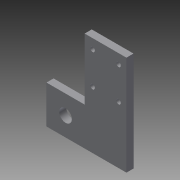
# Autodesk Inventor part: el torro bracket
Saved by Autodesk Inventor 2014 SP1 (Build 180222100, 222)
## iProperties
Created: 2014-02-18
Part Number: el torro bracket
Material: Generic
Document SubType Name: Modeling
Designer: rennoldson eimile
Density: 1 g/cm^3
Appearance: Default
Author: rennoldson eimile
Autodesk Inventor part; units mm, degrees
ref_plane "YZ Plane" through (0, 0, 0) normal (1, 0, 0) x (0, 1, 0)
ref_plane "XZ Plane" through (0, 0, 0) normal (0, 1, 0) x (-1, 0, 0)
ref_plane "XY Plane" through (0, 0, 0) normal (0, 0, 1) x (1, 0, 0)
sketch "Sketch1" plane through (0, 0, 0) normal (0, 0, 1) x (1, 0, 0)
  line L0 (-103.3855, 35.2163) -> (-23.0707, 35.2163)
  line L1 (-23.0707, 35.2163) -> (-23.0707, -64.7835)
  line L2 (-23.0707, -64.7835) -> (-103.3855, -64.7835)
  line L3 (-103.3855, -64.7835) -> (-103.3855, 35.2163)
  dimension "d0" = 80.3148
  dimension "d1" = 99.9998
  constraints: 8 end point, 2 parallel, 1 horizontal, 1 perpendicular
  measures "d0" distance of L1.end L2.end
  measures "d1" distance of L0.end L1.end
extrude "Extrusion1" add sketch "Sketch1" along normal blind 7.1628
sketch "Sketch2" plane through (0, 0, 7.1628) normal (0, 0, 1) x (1, 0, 0)
  line L0 (-23.0707, 35.2163) -> (-103.3855, 35.2163) projected
  line L1 (-103.3855, 35.2163) -> (-103.3855, -64.7835) projected
  line L2 (-103.3855, -64.7835) -> (-23.0707, -64.7835) projected
  line L3 (-23.0707, -64.7835) -> (-23.0707, 35.2163) projected
  line L4 (-65.0315, 35.2163) -> (-65.0315, -26.5819)
  line L5 (-103.3855, -26.5819) -> (-65.0315, -26.5819)
  dimension "d4" = 41.9608
  dimension "d5" = 38.2016
  constraints: 4 end point, 2 point on line, 1 parallel, 1 perpendicular
  measures "d4" distance between parallel lines of L4 L3
  measures "d5" distance between parallel lines of L5 L2
extrude "Extrusion2" cut sketch "Sketch2" against normal blind 7.1628 contours L4 L5 L1 L0
sketch "Sketch3" plane through (0, 0, 7.1628) normal (0, 0, 1) x (1, 0, 0)
  line L0 (-23.0707, 35.2163) -> (-65.0315, 35.2163) projected
  line L1 (-65.0315, -26.5819) -> (-65.0315, -64.7835)
  line L2 (-23.0707, -64.7835) -> (-103.3855, -64.7835) projected
  circle A0 centre (-84.2085, -45.6827) radius 6.35
  dimension "d8" = 12.7
  constraints: 2 end point, 1 centre point, 1 perpendicular, 1 point on line
  measures "d8" diameter of A0
extrude "Extrusion3" cut sketch "Sketch3" against normal blind 7.1628
sketch "Sketch4" plane through (0, 0, 7.1628) normal (0, 0, 1) x (1, 0, 0)
  line L0 (-65.0315, -26.5819) -> (-65.0315, 35.2163) projected
  circle A0 centre (-57.0813, 25.4881) radius 2.3241
  circle A1 centre (-31.0209, 25.4881) radius 2.3241
  circle A2 centre (-57.0813, -7.0239) radius 2.3241
  circle A3 centre (-31.0209, -7.0239) radius 2.3241
  dimension "d15" = 4.6482
  dimension "d16" = 4.6482
  dimension "d17" = 4.6482
  dimension "d18" = 4.6482
  constraints: 4 centre point
  measures "d15" diameter of A0
  measures "d16" diameter of A1
  measures "d17" diameter of A2
  measures "d18" diameter of A3
extrude "Extrusion4" cut sketch "Sketch4" against normal blind 7.1628
body "Solid1"
